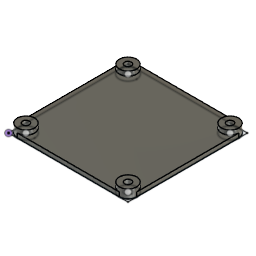
usb_button_interface_base (Autodesk Fusion 360 design; units mm, degrees)
Autodesk Fusion 360 part; units mm, degrees
sketch "Sketch1" plane through (0, 0, 0) normal (0, 0, 1) x (1, 0, 0)
  line L0 (0, 0) -> (55, 0)
  line L1 (55, 0) -> (55, 55)
  line L2 (55, 55) -> (0, 55)
  line L3 (0, 55) -> (0, 0)
  circle A0 centre (4, 51) radius 4
  circle A1 centre (51, 51) radius 4
  circle A2 centre (4, 4) radius 4
  circle A3 centre (51, 4) radius 4
  circle A4 centre (4, 51) radius 1.55
  circle A5 centre (51, 51) radius 1.55
  circle A6 centre (4, 4) radius 1.55
  circle A7 centre (51, 4) radius 1.55
  dimension "d1" = 55
  dimension "d2" = 55
  dimension "d3" = 8
  dimension "d4" = 8
  dimension "d5" = 8
  dimension "d6" = 8
  dimension "d7" = 4
  dimension "d8" = 4
  dimension "d9" = 4
  dimension "d10" = 4
  dimension "d11" = 4
  dimension "d12" = 4
  dimension "d13" = 4
  dimension "d14" = 4
  dimension "d15" = 3.1
  dimension "d16" = 3.1
  dimension "d17" = 3.1
  dimension "d18" = 3.1
  constraint horizontal L0
  constraint vertical L1
  constraint horizontal L2
  constraint vertical L3
  constraint coincident L0.start L3.end
  constraint concentric A0 A4
  constraint concentric A1 A5
  constraint concentric A2 A6
  constraint concentric A3 A7
  measures "d1" distance of L0.start L0.end
  measures "d2" distance of L0.start L2.end
  measures "d3" diameter of A0
  measures "d4" diameter of A1
  measures "d5" diameter of A2
  measures "d6" diameter of A3
  measures "d7" distance of L3 A0.centre
  measures "d8" distance of L2 A0.centre
  measures "d9" distance of L2 A1.centre
  measures "d10" distance of L1 A1.centre
  measures "d11" distance of L3 A2.centre
  measures "d12" distance of L0 A2.centre
  measures "d13" distance of L0 A3.centre
  measures "d14" distance of L1 A3.centre
  measures "d15" diameter of A4
  measures "d16" diameter of A5
  measures "d17" diameter of A6
  measures "d18" diameter of A7
extrude "Extrude1" add sketch "Sketch1" along normal blind 2 contours L0 L1 L2 L3 A0 A1 A2 A3
extrude "Extrude2" add sketch "Sketch1" along normal blind 4 contours A2 | A3 | A0 | A1
chamfer "Chamfer1" distance 1.8 angle 45 4 edges at (2.5549, 4.5605, 0) (49.5549, 4.5605, 0) (49.5549, 51.5605, 0) (2.5549, 51.5605, 0)
